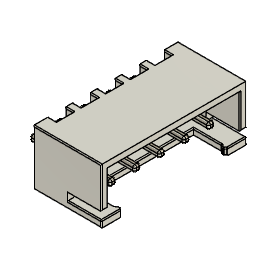
Male_5 (Autodesk Fusion 360 design; units mm, degrees)
Autodesk Fusion 360 part; units mm, degrees
note: some values were not read from the file. Chosen so that the rebuilt part matches the saved one: which pieces of a blend or face edit are solid.
sketch "Sketch1" plane through (0, 0, 0) normal (0, 0, 1) x (1, 0, 0)
  line L0 (3.5, -7.5) -> (-3.5, -7.5)
  line L1 (-3.5, -7.5) -> (-3.5, 7.5)
  line L2 (-3.5, 7.5) -> (3.5, 7.5)
  line L3 (3.5, 7.5) -> (3.5, -7.5)
  line L4 (3.5, -7.5) -> (-3.5, 7.5) construction
  line L5 (-3.5, -7.5) -> (3.5, 7.5) construction
  dimension "d1" = 7
  dimension "d2" = 15
  constraint horizontal L0
  constraint perpendicular L0 L1
  constraint parallel L0 L2
  constraint parallel L1 L3
  constraint coincident L4 origin
  constraint coincident L5 origin
  measures "d1" distance of L1.end L2.end
  measures "d2" distance of L0.end L1.end
extrude "Extrude1" add sketch "Sketch1" along normal blind 5.7
sketch "Sketch2" plane through (3.5, 0, 0) normal (1, 0, 0) x (0, 1, 0)
  line L0 (-7.5, 0) -> (7.5, 0)
  line L1 (7.5, 0) -> (7.5, 5.7)
  line L2 (7.5, 5.7) -> (-7.5, 5.7)
  line L3 (-7.5, 5.7) -> (-7.5, 0)
  line L4 (-6.8, 0.7) -> (6.8, 0.7)
  line L5 (6.8, 0.7) -> (6.8, 5)
  line L6 (6.8, 5) -> (-6.8, 5)
  line L7 (-6.8, 5) -> (-6.8, 0.7)
  dimension "d5" = -0.7
extrude "Extrude2" cut sketch "Sketch2" against normal blind 5.5 contours L4 L5 L6 L7
sketch "Sketch3" plane through (3.5, 0, 0) normal (1, 0, 0) x (0, 1, 0)
  line L0 (6.8, 0.7) -> (-6.8, 0.7)
  line L1 (-6.8, 0.7) -> (-6.8, 5)
  line L2 (-6.8, 5) -> (6.8, 5)
  line L3 (6.8, 5) -> (6.8, 0.7)
  line L4 (-7.5, 0) -> (7.5, 0)
  line L5 (7.5, 0) -> (7.5, 5.7)
  line L6 (7.5, 5.7) -> (-7.5, 5.7)
  line L7 (-7.5, 5.7) -> (-7.5, 0)
  line L8 (-6.8, 0.7) -> (-7.5, 0.7)
  line L9 (-7.5, 1.5) -> (-6.8, 1.5)
  dimension "d8" = 0.8
  constraint coincident L0.end L1.start
  constraint coincident L7 L8.end
  constraint perpendicular L7 L8
  constraint coincident L7 L9.start
  constraint coincident L1 L9.end
  constraint perpendicular L1 L9
  measures "d8" distance of L8 L9
extrude "Extrude3" cut sketch "Sketch3" against normal blind 3.5 contours L1 L7 L8 L9
mirror "Mirror1" about plane through (0, 0, 0) normal (0, 1, 0) of "Extrude3"
sketch "Sketch4" plane through (0, 0, 0) normal (0, 0, -1) x (1, 0, 0)
  line L0 (-3.5, -7.5) -> (3.5, -7.5)
  line L1 (3.5, -7.5) -> (3.5, 7.5)
  line L2 (3.5, 7.5) -> (-3.5, 7.5)
  line L3 (-3.5, 7.5) -> (-3.5, -7.5)
  line L4 (3.5, -7.5) -> (-3.5, -7.5)
  line L5 (-3.5, -7.5) -> (-3.5, -5.5)
  line L6 (-3.5, -5.5) -> (3.5, -5.5)
  line L7 (3.5, -5.5) -> (3.5, -7.5)
  line L8 (3.5, -5.5) -> (2.9, -5.5)
  line L9 (2.9, -5.5) -> (2.9, -5.3)
  line L10 (2.9, -5.3) -> (3.5, -5.3)
  line L11 (3.5, -5.3) -> (3.5, -5.5)
  line L12 (20, 0) -> (2.5, 0)
  line L13 (3.5, 5.5) -> (3.5, 7.5)
  line L14 (3.5, 5.3) -> (3.5, 5.5)
  line L15 (2.9, 5.3) -> (3.5, 5.3)
  line L16 (3.5, 5.5) -> (2.9, 5.5)
  line L17 (2.9, 5.5) -> (2.9, 5.3)
  line L18 (-3.5, 5.5) -> (3.5, 5.5)
  line L19 (3.5, 7.5) -> (-3.5, 7.5)
  line L20 (-3.5, 7.5) -> (-3.5, 5.5)
  line L21 (-3.5, -5.5) -> (0, -5.5)
  line L22 (0, -5.5) -> (0, 5.5)
  line L23 (0, 5.5) -> (-3.5, 5.5)
  line L24 (-3.5, 5.5) -> (-3.5, -5.5)
  line L25 (0, -5.5) -> (0, -4)
  line L26 (0, -4) -> (3.5, -4)
  line L27 (3.5, -4) -> (3.5, -3.9)
  line L28 (3.5, -3.9) -> (0, -3.9)
  line L29 (0, -3.9) -> (0, -4)
  dimension "d13" = 2
  dimension "d14" = 0.6
  dimension "d15" = 0.2
  dimension "d42" = 1.5
  dimension "d43" = 0.1
  constraint horizontal L4
  constraint vertical L5
  constraint horizontal L6
  constraint vertical L7
  constraint coincident L3 L5.end
  constraint coincident L0.end L1.start
  constraint horizontal L8
  constraint vertical L9
  constraint horizontal L10
  constraint vertical L11
  constraint symmetric L0.end L12 L1.end
  constraint symmetric L0.start L12 L2.end
  constraint symmetric L5.end L12 L18.start
  constraint symmetric L6.end L12 L13.start
  constraint symmetric L8.end L12 L16.end
  constraint symmetric L9.end L12 L15.start
  constraint symmetric L10.end L12 L14.start
  constraint horizontal L21
  constraint vertical L22
  constraint horizontal L23
  constraint vertical L24
  constraint midpoint L18 L22.end
  constraint perpendicular L6 L25
  constraint horizontal L26
  constraint vertical L27
  constraint horizontal L28
  constraint vertical L29
  constraint coincident L1 L27.end
  measures "d13" distance of L0.end L6.end
  measures "d14" distance of L6.end L8.end
  measures "d15" distance of L6.end L10.end
  measures "d42" distance of L21.end L25.end
  measures "d43" distance of L25.end L28.end
extrude "Extrude4" cut sketch "Sketch4" against normal blind 1.5 contours L1 L6 L9 L10 L22 L25 L26 | L1 L15 L17 L18 L22 L28 | L1 L22 L26 L27 L28 L29
chamfer "Chamfer1" distance 0.2 angle 45 4 edges at (3.5, -5.3, 0.35) (2.9, -5.3, 0.35) (2.9, 5.3, 0.35) (3.5, 5.3, 0.35)
sketch "Sketch5" plane through (-3.5, 0, 0) normal (-1, 0, 0) x (0, -1, 0)
  line L0 (-7.5, 0) -> (7.5, 0)
  line L1 (7.5, 0) -> (7.5, 5.7)
  line L2 (7.5, 5.7) -> (-7.5, 5.7)
  line L3 (-7.5, 5.7) -> (-7.5, 0)
  line L4 (-5.93, 5.7) -> (-4.23, 5.7)
  line L5 (-4.23, 5.7) -> (-4.23, 0)
  line L6 (-4.23, 0) -> (-5.93, 0)
  line L7 (-5.93, 0) -> (-5.93, 5.7)
  dimension "d19" = 1.7
  dimension "d20" = 1.57
  constraint horizontal L4
  constraint vertical L5
  constraint horizontal L6
  constraint vertical L7
  constraint coincident L0 L5.end
  constraint coincident L2 L4.start
  measures "d19" distance of L5 L7
  measures "d20" distance of L3 L7
extrude "Extrude5" cut sketch "Sketch5" against normal blind 0.8 contours L0 L2 L4 L5 L6 L7
sketch "Sketch6" plane through (-2.7, 0, 0) normal (-1, 0, 0) x (0, -1, 0)
  line L0 (-5.93, 0) -> (-4.23, 0)
  line L1 (-4.23, 0) -> (-4.23, 5.7)
  line L2 (-4.23, 5.7) -> (-5.93, 5.7)
  line L3 (-5.93, 5.7) -> (-5.93, 0)
  line L4 (-4.755, 1.95) -> (-5.405, 1.95)
  line L5 (-5.405, 1.95) -> (-5.405, 2.6)
  line L6 (-5.405, 2.6) -> (-4.755, 2.6)
  line L7 (-4.755, 2.6) -> (-4.755, 1.95)
  line L8 (-4.755, 1.95) -> (-5.405, 2.6) construction
  line L9 (-5.405, 1.95) -> (-4.755, 2.6) construction
  point P0 (-5.08, 2.275)
  dimension "d27" = 0.65
  dimension "d28" = 0.65
  dimension "d29" = 0.85
  dimension "d31" = 2.6
  constraint horizontal L4
  constraint perpendicular L4 L5
  constraint parallel L4 L6
  constraint parallel L5 L7
  constraint coincident L8 P0
  constraint coincident L9 P0
  measures "d27" distance of L5.end L6.end
  measures "d28" distance of L4.end L5.end
  measures "d29" distance of L1 P0
  measures "d31" distance of L0 L6
extrude "Extrude6" add sketch "Sketch6" along normal blind 3.3 contours L4 L5 L6 L7
extrude "Extrude7" add sketch "Sketch6" against normal blind 5 contours L4 L5 L6 L7
fillet "Fillet2" radius 0.2 8 edges at (0.15, 4.755, 1.95) (0.15, 4.755, 2.6) (0.15, 5.405, 1.95) (0.15, 5.405, 2.6) (-4.35, 4.755, 2.6) (-4.35, 4.755, 1.95) (-4.35, 5.405, 2.6) (-4.35, 5.405, 1.95) 2 faces at (2.3, 4.9717, 2.1667) (-6, 4.9717, 2.1667)
fillet "Fillet2" radius 0.1 8 edges at (-3.5, 4.23, 2.85) (-3.5, 5.93, 2.85) (-2.7, 5.08, 5.7) (-3.1, 5.93, 5.7) (-3.1, 4.23, 5.7) (-3.1, 4.23, 0) (-2.7, 5.08, 0) (-3.1, 5.93, 0)
pattern_linear "R-Pattern1" count 5 spacing 2.54 along (0, -1, 0) of "Extrude5", "Extrude6", "Extrude7", "Fillet2"
fillet "Fillet3" radius 0.1 45 edges at (0, 7.5, 5.7) (0, -7.5, 5.7) (0, -7.5, 0) (0, 7.5, 0) (-3.5, -7.5, 2.85) (-3.5, 7.5, 2.85) (3.5, 7.5, 0.35) (3.5, -7.5, 0.35) (3.5, -7.15, 1.5) (3.5, 7.15, 1.5) (3.5, 6.8, 3.25) (3.5, 0, 5) (3.5, -6.8, 3.25) (3.5, -7.5, 3.6) (3.5, 7.5, 3.6) (0, 0, 0) (1.45, -5.5, 0) (0, 0, 0.7) (1.45, 5.5, 0.7) (1.45, 5.5, 0) (3.1, 5.3, 0.35) (3.3, 5.3, 0.35) (3.5, 5.5, 0.35) (2.9, 5.5, 0.35) (3.5, -5.5, 0.35) (3.3, -5.3, 0.35) (3.1, -5.3, 0.35) (2.9, -5.5, 0.35) (1.75, -7.5, 0.7) (1.45, -5.5, 0.7) (3.5, -6.5, 0.7) (3.4, -5.4, 0.7) (3.2, -5.3, 0.7) (3, -5.4, 0.7) (3, 5.4, 0.7) (3.4, 5.4, 0.7) (3.2, 5.3, 0.7) (3.5, 6.5, 0.7) (1.75, 7.5, 0.7) (3, -5.4, 0) (3.2, -5.3, 0) (3.4, -5.4, 0) (3, 5.4, 0) (3.2, 5.3, 0) (3.4, 5.4, 0)
equation "d2 = lengthBasedOnPins"
equation "d20 = spacingBasedOnPins"
equation "d23 = pins"
equation "pins = 5"
equation "lengthBasedOnPins = if(pins == 2; 7.4 mm; if(pins == 3; 10 mm; if(pins == 4; 12.4 mm; if(pins == 5; 15 mm; if(pins == 6; 17.4 mm; 0 mm)))))"
equation "spacingBasedOnPins = if(pins == 2; 1.58 mm; if(pins == 3; 1.61 mm; if(pins == 4; 1.54 mm; if(pins == 5; 1.57 mm; if(pins == 6; 1.50 mm; 0 mm)))))"
named bodies: "Male_5"
